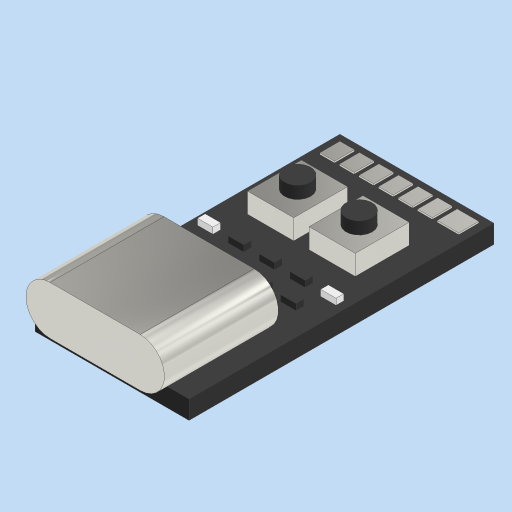
# Autodesk Inventor part: OMGUSB
Saved by Autodesk Inventor 2024 (Build 280153000, 153)
## iProperties
Created: 2025-03-26
Part Number: OMGUSB
Material: Generic
Document SubType Name: Modeling
Designer: XxPan
Density: 1 g/cm^3
Appearance: Default
Author: XxPan
Autodesk Inventor part; units mm, degrees
ref_plane "YZ Plane" through (0, 0, 0) normal (1, 0, 0) x (0, 1, 0)
ref_plane "XZ Plane" through (0, 0, 0) normal (0, 1, 0) x (-1, 0, 0)
ref_plane "XY Plane" through (0, 0, 0) normal (0, 0, 1) x (1, 0, 0)
sketch "Sketch1" plane through (0, 0, 0) normal (0, 0, 1) x (1, 0, 0)
  line L0 (-4.5, 0) -> (4.5, 0) construction
  line L1 (-2.925, -1.575) -> (2.925, -1.575)
  line L2 (2.925, 1.575) -> (-2.925, 1.575)
  arc A0 (-2.925, 1.575) -> (-2.925, -1.575) centre (-2.925, 0) ccw
  arc A1 (2.925, -1.575) -> (2.925, 1.575) centre (2.925, 0) ccw
  point P0 (0, 0)
  point P1 (0, 0)
  dimension "d0" = 9
  dimension "d1" = 3.15
  constraints: 8 end point, 6 point on circle, 4 tangent, 2 centre point, 2 point on line, 1 coincident, 1 horizontal, 1 midpoint, 1 parallel
  measures "d0" distance of L0.start L0.end
  measures "d1" diameter of A1
extrude "Extrusion1" add sketch "Sketch1" against normal blind 7.4
sketch "Sketch2" plane through (-2.925, -1.575, 0) normal (0, -1, 0) x (1, 0, 0)
  line L0 (7.925, -1.1) -> (-2.075, -1.1)
  line L1 (-2.075, -1.1) -> (-2.075, -20.9)
  line L2 (-2.075, -20.9) -> (7.925, -20.9)
  line L3 (7.925, -20.9) -> (7.925, -1.1)
  line L4 (0, 0) -> (5.85, 0) projected
  point P0 (2.925, 0)
  point P1 (2.925, 0)
  point P2 (2.925, -1.1)
  dimension "d4" = 10
  dimension "d5" = 19.8
  dimension "d6" = 1.1
  constraints: 8 end point, 2 midpoint, 2 parallel, 1 horizontal, 1 perpendicular, 1 vertical alignment
  measures "d4" distance of L2.end L1.end
  measures "d5" distance of L1.end L0.end
  measures "d6" distance between parallel lines of L4 L0
extrude "Extrusion2" add sketch "Sketch2" along normal blind 1.2
sketch "Sketch3" plane through (-2.925, -1.575, 0) normal (0, 1, 0) x (1, 0, 0)
  line L0 (-0.575, 9.55) -> (0.425, 9.55)
  line L1 (0.425, 9.55) -> (0.425, 10.05)
  line L2 (0.425, 10.05) -> (-0.575, 10.05)
  line L3 (-0.575, 10.05) -> (-0.575, 9.55)
  line L4 (1.425, 9.55) -> (2.425, 9.55)
  line L5 (2.425, 9.55) -> (2.425, 10.05)
  line L6 (2.425, 10.05) -> (1.425, 10.05)
  line L7 (1.425, 10.05) -> (1.425, 9.55)
  line L8 (3.425, 9.55) -> (4.425, 9.55)
  line L9 (4.425, 9.55) -> (4.425, 10.05)
  line L10 (4.425, 10.05) -> (3.425, 10.05)
  line L11 (3.425, 10.05) -> (3.425, 9.55)
  line L12 (5.425, 9.55) -> (6.425, 9.55)
  line L13 (6.425, 9.55) -> (6.425, 10.05)
  line L14 (6.425, 10.05) -> (5.425, 10.05)
  line L15 (5.425, 10.05) -> (5.425, 9.55)
  line L16 (-2.075, 20.9) -> (7.925, 20.9) projected
  line L17 (2.925, 20.9) -> (2.925, 7.4) construction
  line L18 (5.85, 7.4) -> (0, 7.4) projected
  line L19 (0.425, 11.15) -> (1.425, 11.15)
  line L20 (1.425, 11.15) -> (1.425, 11.65)
  line L21 (1.425, 11.65) -> (0.425, 11.65)
  line L22 (0.425, 11.65) -> (0.425, 11.15)
  line L23 (3.425, 11.15) -> (3.425, 11.65)
  line L24 (3.425, 11.65) -> (2.425, 11.65)
  line L25 (2.425, 11.65) -> (2.425, 11.15)
  line L26 (2.425, 11.15) -> (3.425, 11.15)
  line L27 (5.425, 11.15) -> (5.425, 11.65)
  line L28 (5.425, 11.65) -> (4.425, 11.65)
  line L29 (4.425, 11.65) -> (4.425, 11.15)
  line L30 (4.425, 11.15) -> (5.425, 11.15)
  point P0 (2.925, 0)
  point P1 (-0.575, 9.8)
  point P2 (2.925, 11.65)
  point P3 (0.425, 11.4)
  dimension "d9" = 1
  dimension "d10" = 0.5
  dimension "d13" = 2
  dimension "d18" = 2.4
  dimension "d19" = 1
  dimension "d20" = 0.5
  dimension "d23" = 2
  dimension "d28" = 4
  constraints: 58 end point, 5 midpoint, 4 horizontal, 4 parallel, 2 collinear, 2 perpendicular, 1 point on line, 39 other
  measures "d9" distance of L2.end L1.end
  measures "d10" distance of L1.end L0.end
  measures "d13" distance of L0.start L4.start
  measures "d18" distance from line of L18 point (-0.575, 9.8)
  measures "d19" distance of L21.end L20.end
  measures "d20" distance of L20.end L19.end
  measures "d23" distance of L19.end L23.start
  measures "d28" distance from line of point (0.425, 11.4) L18
extrude "Extrusion3" add sketch "Sketch3" along normal blind 0.4
sketch "Sketch4" plane through (-2.925, -1.575, 0) normal (0, 1, 0) x (1, 0, 0)
  line L0 (-1.575, 11.15) -> (-0.575, 11.15)
  line L1 (-0.575, 11.15) -> (-0.575, 11.65)
  line L2 (-0.575, 11.65) -> (-1.575, 11.65)
  line L3 (-1.575, 11.65) -> (-1.575, 11.15)
  line L4 (6.425, 11.15) -> (7.425, 11.15)
  line L5 (7.425, 11.15) -> (7.425, 11.65)
  line L6 (7.425, 11.65) -> (6.425, 11.65)
  line L7 (6.425, 11.65) -> (6.425, 11.15)
  line L8 (0.425, 11.15) -> (1.425, 11.15) projected
  line L9 (4.425, 11.65) -> (4.425, 11.15) projected
  line L10 (0.425, 11.65) -> (0.425, 11.15) projected
  point P0 (2.925, 0)
  dimension "d31" = 1
  dimension "d32" = 0.5
  dimension "d33" = 1
  dimension "d34" = 0.5
  dimension "d35" = 2
  dimension "d36" = 2
  constraints: 16 end point, 4 parallel, 2 horizontal, 2 perpendicular, 1 collinear, 1 point on line
  measures "d31" distance of L2.end L1.end
  measures "d32" distance of L1.end L0.end
  measures "d33" distance of L6.end L5.end
  measures "d34" distance of L5.end L4.end
  measures "d35" distance between parallel lines of L9 L7
  measures "d36" distance between parallel lines of L3 L10
extrude "Extrusion4" add sketch "Sketch4" along normal blind 0.4
sketch "Sketch5" plane through (-2.925, -1.575, 0) normal (0, 1, 0) x (1, 0, 0)
  line L0 (-0.575, 13.4) -> (2.425, 13.4)
  line L1 (2.425, 13.4) -> (2.425, 16.9)
  line L2 (2.425, 16.9) -> (-0.575, 16.9)
  line L3 (-0.575, 16.9) -> (-0.575, 13.4)
  line L4 (3.425, 13.4) -> (6.425, 13.4)
  line L5 (6.425, 13.4) -> (6.425, 16.9)
  line L6 (6.425, 16.9) -> (3.425, 16.9)
  line L7 (3.425, 16.9) -> (3.425, 13.4)
  line L8 (-2.075, 20.9) -> (7.925, 20.9) projected
  line L9 (5.85, 7.4) -> (0, 7.4) projected
  line L10 (2.925, 7.4) -> (2.925, 20.9) construction
  point P0 (2.925, 0)
  dimension "d39" = 3
  dimension "d40" = 3.5
  dimension "d43" = 4
  dimension "d48" = 4
  constraints: 18 end point, 2 horizontal, 2 midpoint, 2 parallel, 1 collinear, 1 perpendicular, 8 other
  measures "d39" distance of L2.end L1.end
  measures "d40" distance of L1.end L0.end
  measures "d43" distance of L0.start L4.start
  measures "d48" distance between parallel lines of L8 L2
extrude "Extrusion5" add sketch "Sketch5" along normal blind 1.3
sketch "Sketch6" plane through (-2.925, -0.275, 0) normal (0, 1, 0) x (1, 0, 0)
  circle A0 centre (0.925, 15.15) radius 0.85
  circle A1 centre (4.925, 15.15) radius 0.85
  line L0 (-0.575, 16.9) -> (-0.575, 13.4) projected
  line L1 (-0.575, 13.4) -> (2.425, 13.4) projected
  line L2 (3.425, 13.4) -> (6.425, 13.4) projected
  point P0 (2.925, 0)
  point P1 (-0.575, 15.15)
  point P2 (0.925, 13.4)
  point P3 (4.925, 13.4)
  dimension "d51" = 1.7
  dimension "d52" = 1.7
  constraints: 3 midpoint, 2 centre point, 2 horizontal alignment, 2 vertical alignment
  measures "d51" diameter of A0
  measures "d52" diameter of A1
extrude "Extrusion6" add sketch "Sketch6" along normal blind 0.8
sketch "Sketch7" plane through (-2.925, -1.575, 0) normal (0, 1, 0) x (1, 0, 0)
  line L0 (-0.635, 19.11) -> (-1.585, 19.11)
  line L1 (-1.585, 19.11) -> (-1.585, 20.41)
  line L2 (-1.585, 20.41) -> (-0.635, 20.41)
  line L3 (-0.635, 20.41) -> (-0.635, 19.11)
  line L4 (0.635, 19.11) -> (-0.315, 19.11)
  line L5 (-0.315, 19.11) -> (-0.315, 20.41)
  line L6 (-0.315, 20.41) -> (0.635, 20.41)
  line L7 (0.635, 20.41) -> (0.635, 19.11)
  line L8 (1.905, 19.11) -> (0.955, 19.11)
  line L9 (0.955, 19.11) -> (0.955, 20.41)
  line L10 (0.955, 20.41) -> (1.905, 20.41)
  line L11 (1.905, 20.41) -> (1.905, 19.11)
  line L12 (3.175, 19.11) -> (2.225, 19.11)
  line L13 (2.225, 19.11) -> (2.225, 20.41)
  line L14 (2.225, 20.41) -> (3.175, 20.41)
  line L15 (3.175, 20.41) -> (3.175, 19.11)
  line L16 (4.445, 19.11) -> (3.495, 19.11)
  line L17 (3.495, 19.11) -> (3.495, 20.41)
  line L18 (3.495, 20.41) -> (4.445, 20.41)
  line L19 (4.445, 20.41) -> (4.445, 19.11)
  line L20 (5.715, 19.11) -> (4.765, 19.11)
  line L21 (4.765, 19.11) -> (4.765, 20.41)
  line L22 (4.765, 20.41) -> (5.715, 20.41)
  line L23 (5.715, 20.41) -> (5.715, 19.11)
  line L24 (6.985, 19.11) -> (6.035, 19.11)
  line L25 (6.035, 19.11) -> (6.035, 20.41)
  line L26 (6.035, 20.41) -> (6.985, 20.41)
  line L27 (6.985, 20.41) -> (6.985, 19.11)
  line L28 (6.985, 20.41) -> (7.435, 20.41)
  line L29 (7.435, 20.41) -> (7.435, 19.11)
  line L30 (7.435, 19.11) -> (6.985, 19.11)
  line L31 (7.925, 20.9) -> (7.925, 1.1) projected
  line L32 (-2.075, 1.1) -> (-2.075, 20.9) projected
  line L33 (-2.075, 20.9) -> (7.925, 20.9) projected
  point P0 (2.925, 0)
  dimension "d55" = 0.95
  dimension "d56" = 1.3
  dimension "d59" = 1.27
  dimension "d64" = 1.4
  dimension "d65" = 10
  dimension "d66" = 9.02
  dimension "d67" = 0.49
  dimension "d68" = 0.49
  constraints: 62 end point, 3 horizontal, 3 perpendicular, 2 parallel, 1 collinear, 47 other
  measures "d55" distance of L1.end L2.end
  measures "d56" distance of L0.end L1.end
  measures "d59" distance of L0.start L4.start
  measures "d64" distance between parallel lines of L25 L29
  measures "d65" distance between parallel lines of L32 L31
  measures "d66" distance between parallel lines of L1 L29
  measures "d67" distance between parallel lines of L29 L31
  measures "d68" distance between parallel lines of L2 L33
extrude "Extrusion7" add sketch "Sketch7" along normal blind 0.1 and the other way blind 1.4
equation "\"d67\" = -0.5 * d66 + 0.5 * d65"
equation "\"d68\" = d67"
body "Solid1"
